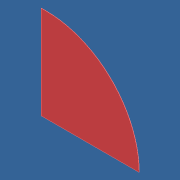
# Autodesk Inventor part: GE-12050
Saved by Autodesk Inventor 2012 (Build 160160000, 160)
## iProperties
Created: 2011-08-26
Part Number: GE-12050
Document SubType Name: Modeling
Designer: mcyr
Density: 1 g/cm^3
Description: Key Plastic
Material: Default
Title: Key Plastic
Author: mcyr
Autodesk Inventor part; units mm, degrees
ref_plane "YZ Plane" through (0, 0, 0) normal (1, 0, 0) x (0, 1, 0)
ref_plane "XZ Plane" through (0, 0, 0) normal (0, 1, 0) x (-1, 0, 0)
ref_plane "XY Plane" through (0, 0, 0) normal (0, 0, 1) x (1, 0, 0)
sketch "Sketch1" plane through (0, 0, 0) normal (0, 0, 1) x (1, 0, 0)
  line L0 (0, 0) -> (0, 1219.2)
  line L1 (0, 0) -> (1282.7, 0)
  line L2 (0, 1219.2) -> (63.5, 1219.2)
  arc A0 (1282.7, 0) -> (63.5, 1219.2) centre (63.5, 0) ccw
  dimension "d0" = 1219.2
  dimension "d1" = 1282.7
  dimension "d5" = 63.5
  dimension "d6" = 1219.2
  constraints: 6 end point, 2 point on circle, 1 centre point, 1 parallel, 1 perpendicular, 1 vertical
  measures "d0" distance of L0.start L0.end
  measures "d1" distance of L0.start L1.end
  measures "d5" distance of L0.end L2.end
  measures "d6" radius of A0
extrude "Extrusion1" add sketch "Sketch1" along normal blind 3.175
body "Solid1"
